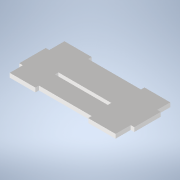
# Autodesk Inventor part: Platte3-Seite
Saved by Autodesk Inventor 2020.3 (Build 243373010, 373A)
## iProperties
Created: 2020-11-28
Part Number: Platte3-Seite
Material: Generisch
Document SubType Name: Modeling
Designer: Stefan
Density: 1 g/cm^3
Appearance: Vorgabe
Author: Stefan
Autodesk Inventor part; units mm, degrees
ref_plane "YZ Plane" through (0, 0, 0) normal (1, 0, 0) x (0, 1, 0)
ref_plane "XZ Plane" through (0, 0, 0) normal (0, 1, 0) x (-1, 0, 0)
ref_plane "XY Plane" through (0, 0, 0) normal (0, 0, 1) x (1, 0, 0)
sketch "Skizze1" plane through (0, 0, 0) normal (0, 1, 0) x (-1, 0, 0)
  line L0 (-106.0247, -103.5796) -> (-106.0247, -93.5796)
  line L1 (-106.0247, -93.5796) -> (43.9753, -93.5796)
  line L2 (43.9753, -93.5796) -> (43.9753, -103.5796)
  line L3 (-178.9745, -103.5796) -> (-106.0247, -103.5796)
  line L4 (43.9753, -103.5796) -> (121.0255, -103.5796)
  line L5 (-101.4396, 51.4204) -> (-101.4396, 41.4204)
  line L6 (-101.4396, 41.4204) -> (48.5604, 41.4204)
  line L7 (48.5604, 41.4204) -> (48.5604, 51.4204)
  line L8 (121.0255, 51.4204) -> (48.5604, 51.4204)
  line L9 (-101.4396, 51.4204) -> (-178.9119, 51.4204)
  line L10 (121.0255, 11.4204) -> (131.0255, 11.4204)
  line L11 (131.0255, 11.4204) -> (131.0255, -63.5796)
  line L12 (131.0255, -63.5796) -> (121.0255, -63.5796)
  line L13 (121.0255, -103.5796) -> (121.0255, -63.5796)
  line L14 (121.0255, 11.4204) -> (121.0255, 51.4204)
  line L15 (53.134, -8.5796) -> (-96.866, -8.5796)
  line L16 (-96.866, -8.5796) -> (-96.866, -18.5796)
  line L17 (-96.866, -18.5796) -> (53.134, -18.5796)
  line L18 (53.134, -18.5796) -> (53.134, -8.5796)
  line L19 (-178.9119, 11.4204) -> (-188.9745, 11.4204)
  line L20 (-188.9745, 11.4204) -> (-188.9745, -63.5796)
  line L21 (-188.9745, -63.5796) -> (-178.9745, -63.5796)
  line L22 (-178.9119, 51.4204) -> (-178.9119, 11.4204)
  line L23 (-178.9745, -63.5796) -> (-178.9745, -103.5796)
  point P0 (0, 0)
  dimension "d0" = 300
  dimension "d2" = 150
  dimension "d3" = 10
  dimension "d5" = 150
  dimension "d6" = 10
  dimension "d7" = 10
  dimension "d8" = 75
  dimension "d10" = 150
  dimension "d11" = 10
  dimension "d13" = 10
  dimension "d14" = 75
  dimension "d17" = 10
  dimension "d20" = 10
  dimension "d22" = 50
  dimension "d23" = 0
  dimension "d25" = 155
  dimension "d26" = 0
  dimension "d27" = 10
  dimension "d28" = 40
  dimension "d29" = 40
  constraints: 48 end point, 14 parallel, 7 perpendicular, 5 horizontal
  measures "d0" distance of L4.end L3.start
  measures "d2" distance of L0.end L1.end
  measures "d3" distance of L0.start L0.end
  measures "d5" distance of L6.end L5.end
  measures "d6" distance of L5.end L5.start
  measures "d7" distance of L11.end L12.end
  measures "d8" distance of L10.end L11.end
  measures "d10" distance of L17.end L16.end
  measures "d11" distance of L16.end L15.end
  measures "d13" distance of L21.end L20.end
  measures "d14" distance of L20.end L19.end
  measures "d17" distance between parallel lines of L8 L6
  measures "d20" distance of L1.end L2.end
  measures "d22" distance between parallel lines of L6 L15
  measures "d23" angle of L1 L17
  measures "d25" distance between parallel lines of L3 L9
  measures "d26" horizontal distance of L7.end L6.end
  measures "d27" distance of L10.start L10.end
  measures "d28" distance between parallel lines of L4 L12
  measures "d29" distance between parallel lines of L3 L21
extrude "Extrusion1" add sketch "Skizze1" along normal blind 12
